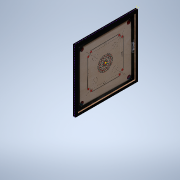
# Autodesk Inventor part: S.Carrom board
Saved by Autodesk Inventor 2020 (Build 240168000, 168)
## iProperties
Created: 2015-04-24
Part Number: S.Carrom board
Material: Birch
Document SubType Name: Modeling
Designer: sandeep suddarsi
Density: 0.512 g/cm^3
Appearance: Birch - Natural Medium Gloss
Author: sandeep suddarsi
Autodesk Inventor part; units mm, degrees
ref_plane "YZ Plane" through (0, 0, 0) normal (1, 0, 0) x (0, 1, 0)
ref_plane "XZ Plane" through (0, 0, 0) normal (0, 1, 0) x (-1, 0, 0)
ref_plane "XY Plane" through (0, 0, 0) normal (0, 0, 1) x (1, 0, 0)
sketch "Sketch1" plane through (0, 0, 0) normal (1, 0, 0) x (0, 1, 0)
  line L0 (250, 250) -> (-250, 250)
  line L1 (-250, 250) -> (-250, -250)
  line L2 (-250, -250) -> (250, -250)
  line L3 (250, -250) -> (250, 250)
  line L4 (250, 250) -> (-250, -250) construction
  line L5 (-250, 250) -> (250, -250) construction
  point P0 (0, 0)
  dimension "d0" = 500
  dimension "d1" = 500
  constraints: 12 end point, 2 midpoint, 2 parallel, 1 horizontal, 1 perpendicular
  measures "d0" distance of L1.end L2.end
  measures "d1" distance of L2.end L0.start
extrude "Extrusion1" add sketch "Sketch1" along normal blind 10
sketch "Sketch2" plane through (10, 0, 0) normal (1, 0, 0) x (0, 0, -1)
  line L0 (-250, 250) -> (-250, -250) projected
  line L1 (-250, -250) -> (250, -250) projected
  line L2 (250, -250) -> (250, 250) projected
  line L3 (250, 250) -> (-250, 250) projected
  line L4 (-230, 230) -> (230, 230)
  line L5 (230, 230) -> (230, -230)
  line L6 (230, -230) -> (-230, -230)
  line L7 (-230, -230) -> (-230, 230)
  line L8 (-230, 230) -> (230, -230) construction
  line L9 (230, 230) -> (-230, -230) construction
  point P0 (0, 0)
  dimension "d4" = 20
  dimension "d5" = 20
  constraints: 12 end point, 2 midpoint, 2 parallel, 1 horizontal, 1 perpendicular
  measures "d4" distance between parallel lines of L3 L4
  measures "d5" distance between parallel lines of L0 L7
extrude "Extrusion2" add sketch "Sketch2" along normal blind 10
sketch "Sketch3" plane through (10, 0, 0) normal (1, 0, 0) x (0, 0, -1)
  circle A0 centre (-200, -200) radius 30
  line L0 (-250, 250) -> (-250, -250) projected
  line L1 (-250, -250) -> (250, -250) projected
  point P0 (0, 0)
  dimension "d8" = 60
  dimension "d9" = 50
  dimension "d10" = 50
  constraints: 1 centre point
  measures "d8" diameter of A0
  measures "d9" distance from line of L0 A0.centre
  measures "d10" distance from line of A0.centre L1
hole "Hole1" at (10, -200, 200) direction (-1, 0, 0) diameter 30 depth 67.75
mirror "Mirror1" about plane through (0, 0, 0) normal (0, 1, 0) of "Hole1"
mirror "Mirror2" about plane through (0, 0, 0) normal (0, 0, 1) of "Hole1", "Mirror1"
sketch "Sketch4" plane through (10, 0, 0) normal (1, 0, 0) x (0, 0, -1)
  line L0 (-250, 250) -> (254.1843, 248.5364) construction
  line L1 (254.1843, 248.5364) -> (252.7352, -250.6505) construction
  line L2 (252.7352, -250.6505) -> (-251.4491, -249.1869) construction
  line L3 (-251.4491, -249.1869) -> (-250, 250) construction
  point P0 (0, 0)
  constraints: 2 other
body "Solid1"
